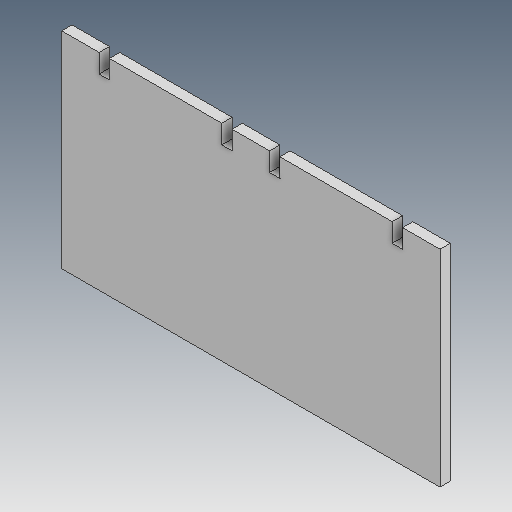
# Autodesk Inventor part: wire_bottom
Saved by Autodesk Inventor 2020 (Build 240168000, 168)
## iProperties
Created: 2021-05-11
Part Number: wire_bottom
Material: Generic
Document SubType Name: Modeling
Designer: Hsu Daniel
Density: 1 g/cm^3
Appearance: Default
Author: Hsu Daniel
Autodesk Inventor part; units mm, degrees
ref_plane "YZ Plane" through (0, 0, 0) normal (1, 0, 0) x (0, 1, 0)
ref_plane "XZ Plane" through (0, 0, 0) normal (0, 1, 0) x (-1, 0, 0)
ref_plane "XY Plane" through (0, 0, 0) normal (0, 0, 1) x (1, 0, 0)
sketch "Sketch2" plane through (0, 0, 0) normal (0, 0, 1) x (1, 0, 0)
  line L0 (0, 0) -> (106.5, 0)
  line L1 (106.5, 0) -> (106.5, 110) construction
  line L2 (106.5, 110) -> (0, 110)
  line L3 (0, 110) -> (0, 0)
  line L4 (213, 0) -> (106.5, 0)
  line L5 (106.5, 110) -> (213, 110)
  line L6 (213, 110) -> (213, 0)
  line L7 (5.5, 100) -> (5.5, 110)
  line L8 (5.5, 110) -> (0, 110)
  line L9 (0, 110) -> (0, 100)
  line L10 (0, 100) -> (5.5, 100)
  line L11 (5.5, 100) -> (0, 110) construction
  line L12 (5.5, 110) -> (0, 100) construction
  line L13 (213, 100) -> (207.5, 100)
  line L14 (207.5, 100) -> (207.5, 110)
  line L15 (207.5, 110) -> (213, 110)
  line L16 (207.5, 100) -> (213, 110) construction
  line L17 (207.5, 110) -> (213, 100) construction
  line L18 (213, 110) -> (213, 100)
  line L19 (106.5, 0.9442) -> (106.5, 183.5442) construction
  line L20 (31, 100) -> (31, 110)
  line L21 (25.5, 110) -> (25.5, 100)
  line L22 (25.5, 100) -> (31, 100)
  line L23 (31, 100) -> (25.5, 110) construction
  line L24 (31, 110) -> (25.5, 100) construction
  line L25 (96.5, 100) -> (96.5, 110)
  line L26 (91, 110) -> (91, 100)
  line L27 (91, 100) -> (96.5, 100)
  line L28 (96.5, 100) -> (91, 110) construction
  line L29 (96.5, 110) -> (91, 100) construction
  line L30 (122, 100) -> (116.5, 100)
  line L31 (116.5, 100) -> (116.5, 110)
  line L32 (116.5, 100) -> (122, 110) construction
  line L33 (116.5, 110) -> (122, 100) construction
  line L34 (122, 110) -> (122, 100)
  line L35 (187.5, 100) -> (182, 100)
  line L36 (182, 100) -> (182, 110)
  line L37 (182, 110) -> (187.5, 100) construction
  line L38 (182, 100) -> (187.5, 110) construction
  line L39 (187.5, 110) -> (187.5, 100)
  line L40 (28.25, 105) -> (93.75, 105) construction
  line L41 (5.5, 100) -> (5.5, 0)
  line L42 (207.5, 100) -> (207.5, 0)
  point P0 (0, 100)
  point P1 (119.25, 105)
  point P2 (184.75, 105)
  point P3 (182, 110)
  point P4 (31, 110)
  point P5 (25.5, 110)
  dimension "d18" = 106.5
  dimension "d19" = 5.5
  dimension "d30" = 10
  dimension "d33" = 100
  dimension "d38" = 10
  dimension "d47" = 20
  constraints: 86 end point, 16 symmetric about line, 9 midpoint, 7 collinear, 6 parallel, 4 perpendicular, 4 point on line, 3 horizontal, 2 coincident, 1 vertical
  measures "d18" distance of L5.start L3.start
  measures "d19" distance of L8.end L7.end
  measures "d30" distance of L7.start L7.end
  measures "d33" distance between parallel lines of L0 L10
  measures "d38" distance between parallel lines of L19 L25
  measures "d47" distance between parallel lines of L7 L21
extrude "Extrusion3" add sketch "Sketch2" along normal blind 5.5 contours L41 L7 L2 L21 L22 L20 L26 L27 L25 L5 L31 L30 L34 L36 L35 L39 L14 L42 L4 L0
equation "\"d38\" = 0.5 * d43"
equation "\"d47\" = lrbottomw"
equation "\"thick\" = 0.5"
equation "\"lrlr\" = 19"
equation "\"lrmid\" = 19.9"
equation "\"lrdepth\" = 3.3"
equation "\"mlr\" = 16.6"
equation "\"mmid\" = 24.7"
equation "\"mdepth\" = 4.5"
equation "\"lrltotal\" = 126.6"
equation "\"mltotal\" = 126.6"
equation "\"lrbetween\" = 52.1"
equation "\"mbetween\" = 49.5"
equation "\"toler\" = 1"
equation "\"lrbottomw\" = 20"
equation "\"tight\" = 0.08"
equation "\"stuckw\" = 6"
equation "\"sidewallL\" = 132.6"
equation "\"heaterH\" = 117.3"
equation "\"stickL\" = 3.5"
equation "\"wireH\" = 25"
equation "\"d43\" = 20"
body "Solid3"
